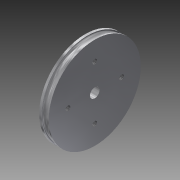
# Autodesk Inventor part: hoiiru
Saved by Autodesk Inventor 2015 (Build 190159000, 159)
## iProperties
Created: 2013-10-28
Part Number: hoiiru
Material: アルミニウム 6061-O
Document SubType Name: Modeling
Designer: kenta
Density: 0.300751 g/cm^3
Appearance: アルミニウム - つや出し
Mass: 2.507 g
Surface Area: 47.5883 cm^2
Volume: 8.33581 cm^3
Author: kenta
Autodesk Inventor part; units mm, degrees
ref_plane "YZ Plane" through (0, 0, 0) normal (1, 0, 0) x (0, 1, 0)
ref_plane "XZ Plane" through (0, 0, 0) normal (0, 1, 0) x (-1, 0, 0)
ref_plane "XY Plane" through (0, 0, 0) normal (0, 0, 1) x (1, 0, 0)
sketch "スケッチ1" plane through (0, 0, 0) normal (0, 0, 1) x (1, 0, 0)
  line L0 (-2.5294, 6.0706) -> (-2.5294, -17.9294)
  line L1 (-2.5294, -17.9294) -> (-7.5294, -17.9294)
  line L2 (-7.5294, -17.9294) -> (-7.5294, 6.0706)
  arc A0 (-6.2794, 6.0706) -> (-3.2794, 6.0706) centre (-4.7794, 6.0706) ccw
  line L3 (-7.5294, 6.0706) -> (-6.2794, 6.0706)
  line L4 (-3.2794, 6.0706) -> (-2.5294, 6.0706)
  point P0 (0, 0)
  dimension "d0" = 5
  dimension "d3" = 3
  constraints: 10 end point, 3 parallel, 2 horizontal, 2 perpendicular, 2 point on circle, 1 centre point
  measures "d0" distance between parallel lines of L0 L2
  measures "d3" diameter of A0
revolve "回転1" add sketch "スケッチ1" angle 360 about axis through (-2.5294, -17.9294, 0) along (-1, 0, 0)
sketch "スケッチ2" plane through (-2.5294, -17.9294, 0) normal (1, 0, 0) x (0, 0, -1)
  circle A0 centre (0, 0) radius 24 projected
  circle A1 centre (0, 0) radius 14
  circle A2 centre (-14, 0) radius 1.5
  circle A3 centre (14, 0) radius 1.5
  circle A4 centre (0, -14) radius 1.5
  circle A5 centre (0, 14) radius 1.5
  point P0 (0, 17.9294)
  dimension "d5" = 28
  dimension "d7" = 3
  dimension "d8" = 3
  dimension "d9" = 3
  dimension "d10" = 3
  constraints: 5 centre point, 4 point on circle, 1 coincident
  measures "d5" diameter of A1
  measures "d7" diameter of A2
  measures "d8" diameter of A4
  measures "d9" diameter of A3
  measures "d10" diameter of A5
hole "穴1" at (-2.5294, -3.9294, 0) at (-2.5294, -17.9294, 14) at (-2.5294, -31.9294, 0) at (-2.5294, -17.9294, -14) direction (-1, 0, 0) diameter 2.459 end through all thread size "M3x0.5" class "6H" standard "ANSI Metric M Profile"
sketch "スケッチ3" plane through (-2.5294, -17.9294, 0) normal (1, 0, 0) x (0, 0, -1)
  circle A0 centre (0, 0) radius 24 projected
  circle A1 centre (0, 0) radius 2.5
  point P0 (0, 17.9294)
  dimension "d18" = 5
  constraints: 1 centre point, 1 coincident
  measures "d18" diameter of A1
hole "穴2" at (-2.5294, -17.9294, 0) direction (-1, 0, 0) diameter 5 end through all
